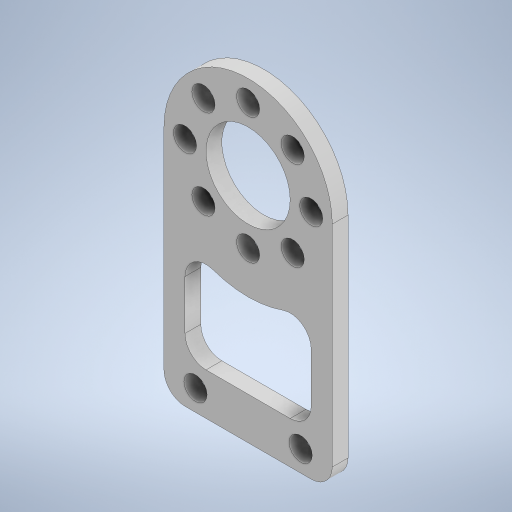
# Autodesk Inventor part: tunage
Saved by Autodesk Inventor 2024 (Build 280153000, 153)
## iProperties
Created: 2024-01-14
Part Number: tunage
Material: 一般
Document SubType Name: Modeling
Designer: right
Density: 1 g/cm^3
Appearance: 既定
Author: right
Autodesk Inventor part; units mm, degrees
ref_plane "YZ Plane" through (0, 0, 0) normal (1, 0, 0) x (0, 1, 0)
ref_plane "XZ Plane" through (0, 0, 0) normal (0, 1, 0) x (-1, 0, 0)
ref_plane "XY Plane" through (0, 0, 0) normal (0, 0, 1) x (1, 0, 0)
sketch "スケッチ1" plane through (0, 0, 0) normal (0, 0, 1) x (1, 0, 0)
  circle A0 centre (0, 0) radius 4
  circle A1 centre (0, 0) radius 6 construction
  circle A2 centre (0, 6) radius 1.1
  circle A3 centre (-4.2426, 4.2426) radius 1.1
  circle A4 centre (-6, 0) radius 1.1
  circle A5 centre (-4.2426, -4.2426) radius 1.1
  circle A6 centre (0, -6) radius 1.1
  circle A7 centre (4.2426, -4.2426) radius 1.1
  circle A8 centre (6, 0) radius 1.1
  circle A9 centre (4.2426, 4.2426) radius 1.1
  circle A10 centre (0, 0) radius 8
  circle A11 centre (-5, -20) radius 1.1
  circle A12 centre (5, -20) radius 1.1
  line L0 (0, 6) -> (0, 0) construction
  line L1 (-8, -22) -> (8, -22)
  line L2 (8, -22) -> (8, -18)
  line L3 (8, -18) -> (-8, -18)
  line L4 (-8, -18) -> (-8, -22)
  line L5 (-8, -22) -> (8, -18) construction
  line L6 (8, -22) -> (-8, -18) construction
  line L7 (-8, 0) -> (-8, -18)
  line L8 (8, 0) -> (8, -18)
  circle A13 centre (0, 0) radius 10
  line L9 (-6, -8) -> (-6, -18)
  line L10 (6, -8) -> (6, -18)
  point P0 (0, -20)
  point P1 (6, -18)
  point P2 (8, 0)
  dimension "d1" = 12
  dimension "d7" = 16
  dimension "d15" = 2
  dimension "d0" = 8
  dimension "d2" = 2.2
  dimension "d5" = 360
  dimension "d8" = 2.2
  dimension "d9" = 2.2
  dimension "d10" = 10
  dimension "d11" = 20
  dimension "d12" = 5
  dimension "d14" = 2
  dimension "d16" = 2
  constraints: 22 end point, 11 centre point, 4 coincident, 4 symmetric about line, 3 horizontal alignment, 3 vertical alignment, 2 midpoint, 2 parallel, 2 perpendicular, 2 vertical, 1 horizontal, 1 point on line, 25 other
  measures "d0" diameter of A0
  measures "d2" diameter of A2
  measures "d8" diameter of A11
  measures "d9" diameter of A12
  measures "d10" distance of A12.centre A11.centre
  measures "d11" vertical distance of A12.centre point (0, 0)
  measures "d12" distance from line of A12.centre L0
  measures "d14" distance from line of L1 A12.centre
  measures "d16" distance between parallel lines of L7 L9
extrude "押し出し1" add sketch "スケッチ1" along normal blind 1.5 contours A10 | L8 A13 L7 A10 | L8 L3 L10 A13 | A13 L9 L3 L7 | L2 L1 L4 L3 picked at (4.9014, -7.8926)
fillet "フィレット1" radius 2 6 edges at (-6, -8, 0.75) (6, -8, 0.75) (-6, -18, 0.75) (6, -18, 0.75) (-8, -22, 0.75) (8, -22, 0.75)
equation "\"d12\" = 0.5 * d10"
equation "\"d16\" = d15"
